Autodesk Fusion 360 part; units mm, degrees
(part 6 of 6)
extrude "Extrude4" add sketch "Sketch1" along normal blind 5 contours L33 L34 L35 L36
equation "d6 = 37.200 mm + 5 mm + 5 mm"
equation "d7 = 10.200 mm + 10 mm"

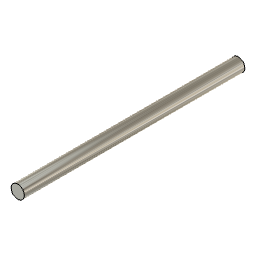
design "50mm rod"
Autodesk Fusion 360 part; units mm, degrees
sketch "Sketch1" plane through (0, 0, 0) normal (0, 1, 0) x (1, 0, 0)
  circle A0 centre (0, 0) radius 1.5
  dimension "d1" = 3
  constraint coincident A0.centre origin
  measures "d1" diameter of A0
extrude "Extrude1" add sketch "Sketch1" along normal blind 50
